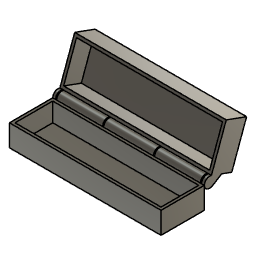
HingedBox (Autodesk Fusion 360 design; units mm, degrees)
part number: 2025-04-19-17-20-53-155
part number: 2025-04-19-17-30-47-805
part number: 2025-04-19-17-34-28-334
Autodesk Fusion 360 part; units mm, degrees
note: some values were not read from the file. Set by a fixed rule: which sketch regions a step uses.
sketch "Sketch1" plane through (0, 0, 0) normal (0, 0, 1) x (1, 0, 0)
  line L0 (0, 0) -> (70, 0)
  line L1 (70, 0) -> (70, 20)
  line L2 (70, 20) -> (0, 20)
  line L3 (0, 20) -> (0, 0)
  dimension "d1" = 70
  dimension "d2" = 20
  constraint horizontal L0
  constraint vertical L1
  constraint horizontal L2
  constraint vertical L3
  constraint coincident L0.start L3.end
  measures "d1" distance of L0.start L0.end
  measures "d2" distance of L0.start L2.end
extrude "Extrude1" add sketch "Sketch1" along normal blind 10 makes body 1
shell "Shell1" thickness 1.3 removed faces 1 at (23.3333, 13.3333, 10) on bodies 1
copy_body "CopyPasteBodies1" bodies 1 makes body 2
move_body "Move1" bodies 2 to x (1, 0, 0) y (0, 1, 0) z (0, 0, 1) at (0, -24.9, 0)
copy_body "CutPasteBodies1" bodies 1 removing the originals makes body 3 in component "box1"
copy_body "CutPasteBodies1'" bodies 2 removing the originals makes body 4 in component "box2"
sketch "Sketch1 (2)" plane through (70, 0, 0) normal (1, 0, 0) x (0, 1, 0) in component "box2"
  line L0 (-24.9, 0) -> (-4.9, 0)
  line L1 (-4.9, 0) -> (-4.9, 10)
  line L2 (-4.9, 10) -> (-24.9, 10)
  line L3 (-24.9, 10) -> (-24.9, 0)
  line L4 (-4.9, 10) -> (-2.45, 10)
  circle A0 centre (-2.45, 10) radius 2.45
  line L5 (-4.9, 5) -> (-0.9487, 8.0639)
  dimension "d10" = 2.45
  constraint coincident L1.end L2.start
  constraint perpendicular L1 L4
  constraint coincident L4.end A0.centre
  constraint coincident L1.end A0
  constraint midpoint L1 L5.start
  constraint coincident A0 L5.end
  constraint tangent A0 L5
  measures "d10" distance of L1.end L4.end
extrude "Extrude1'" add sketch "Sketch1 (2)" along normal blind -22.5 and the other way blind 1.3 from surface at -0.5 contours L1 A0 L5 | A0 picked at (-3.9834, 6.8707) picked at (-1.7866, 9.7088) bodies 4 in component "box2"
sketch "Sketch2" plane through (0, 0, 0) normal (-1, 0, 0) x (0, -1, 0) in component "box2"
  line L0 (4.9, 0) -> (24.9, 0)
  line L1 (24.9, 0) -> (24.9, 10)
  line L2 (24.9, 10) -> (4.9, 10)
  line L3 (4.9, 10) -> (4.9, 0)
  circle A0 centre (2.45, 10) radius 2.452
  line L4 (4.9, 5) -> (0.9482, 8.0616)
  dimension "d13" = 2.45
  constraint midpoint L3 L4.start
  constraint coincident A0 L4.end
  constraint tangent A0 L4
  measures "d13" distance of L2.end A0.centre
extrude "Extrude2" add sketch "Sketch2" along normal blind -22.5 and the other way blind 1.3 from surface at -0.5 contours L3 A0 L4 | L2 L3 A0 picked at (3.9543, 6.8551) picked at (1.637, 10.0477) bodies 4 in component "box2"
hole "Hole1" at (0, -2.45, 10) direction (1, 0, 0) diameter 2.3 depth 23 tip angle 180 bodies 4 in component "box2"
hole "Hole2" at (70, -2.45, 10) direction (-1, 0, 0) diameter 2.3 depth 23 tip angle 180 bodies 4 in component "box2"
move_face "MoveFace1" by (0, 6, 0) 1 faces at (1.8, -2.8232, 7.3082) on bodies 4 in component "box2"
sketch "Sketch1 (3)" plane through (0, 0, 0) normal (-1, 0, 0) x (0, -1, 0) in component "box1"
  line L0 (-20, 0) -> (0, 0)
  line L1 (0, 0) -> (0, 10)
  line L2 (0, 10) -> (-20, 10)
  line L3 (-20, 10) -> (-20, 0)
  circle A0 centre (2.45, 10) radius 2.45
  line L4 (0, 5) -> (3.9513, 8.0639)
  dimension "d22" = 2.45
  constraint midpoint L1 L4.start
  constraint coincident A0 L4.end
  constraint tangent A0 L4
  measures "d22" distance of L1.end A0.centre
extrude "Extrude1''" add sketch "Sketch1 (3)" against normal blind 1.3 contours L1 A0 L4 | A0 picked at (0.9166, 6.8707) picked at (3.0866, 9.8271) bodies 3 in component "box1"
sketch "Sketch2 (2)" plane through (70, 0, 0) normal (1, 0, 0) x (0, 1, 0) in component "box1"
  line L0 (0, 0) -> (20, 0)
  line L1 (20, 0) -> (20, 10)
  line L2 (20, 10) -> (0, 10)
  line L3 (0, 10) -> (0, 0)
  circle A0 centre (-2.45, 10) radius 2.45
  line L4 (0, 5) -> (-3.9513, 8.0639)
  dimension "d25" = 2.45
  constraint midpoint L3 L4.start
  constraint coincident A0 L4.end
  constraint tangent A0 L4
  measures "d25" distance of L2.end A0.centre
extrude "Extrude2'" add sketch "Sketch2 (2)" along normal blind -23.5 and the other way blind 46.5 contours L3 A0 L4 | A0 picked at (-0.9166, 6.8707) picked at (-1.2089, 10.6236) bodies 3 in component "box1"
sketch "Sketch3" plane through (70, 0, 0) normal (1, 0, 0) x (0, 1, 0) in component "box1"
  line L0 (0, 0) -> (20, 0)
  line L1 (20, 0) -> (20, 10)
  line L2 (20, 10) -> (0, 10)
  line L3 (0, 10) -> (0, 0)
  line L4 (0, 10) -> (-2.45, 10)
  circle A0 centre (-2.45, 10) radius 2.45
  line L5 (0, 5) -> (-3.9513, 8.0639)
  dimension "d30" = 2.45
  constraint coincident L2.end L3.start
  constraint perpendicular L3 L4
  constraint coincident L4.end A0.centre
  constraint coincident L2.end A0
  constraint coincident A0 L5.end
  constraint tangent A0 L5
  measures "d30" distance of L2.end L4.end
extrude "Extrude3" add sketch "Sketch3" against normal blind 1.3 contours L3 A0 L5 | A0 picked at (-0.9166, 6.8707) picked at (-1.6888, 9.8416) bodies 3 in component "box1"
hole "Hole1'" at (70, -2.45, 10) direction (-1, 0, 0) diameter 2.3 depth 1.3 tip angle 180 bodies 3 in component "box1"
hole "Hole2'" at (46.5, -2.45, 10) direction (-1, 0, 0) diameter 2.3 depth 23 tip angle 180 bodies 3 in component "box1"
hole "Hole3" at (0, -2.45, 10) direction (1, 0, 0) diameter 2.3 depth 1.3 tip angle 180 bodies 3 in component "box1"
sketch "Sketch4" plane through (68.7, 0, 0) normal (-1, 0, 0) x (0, -1, 0) in component "box1"
  circle A0 centre (2.45, 10) radius 1.15
  arc A1 (3.9513, 8.0639) -> (0, 10) centre (2.45, 10) ccw
  line L0 (0, 10) -> (0, 5)
  line L1 (0, 5) -> (3.9513, 8.0639)
  circle A2 centre (2.45, 10) radius 1.15
  dimension "d48" = 2.45
  dimension "d49" = 2.3
  measures "d48" distance of A1.end A0.centre
  measures "d49" diameter of A2
extrude "Extrude4" add sketch "Sketch4" along normal blind 68.7 and the other way blind 1.3 contours A0 A2 picked at (2.731, 10.375) bodies 3 in component "box1"
move_body "Move1'" bodies 3 to x (1, 0, 0) y (0, 0.34202, 0.939693) z (0, -0.939693, 0.34202) at (0, 7.7849, 8.882) in component "box1"
component "box1" placed x (1, 0, 0) y (0, 1, 0) z (0, 0, 1) at (0, 0, 0)
component "box2" placed x (1, 0, 0) y (0, 1, 0) z (0, 0, 1) at (0, 0, 0)
